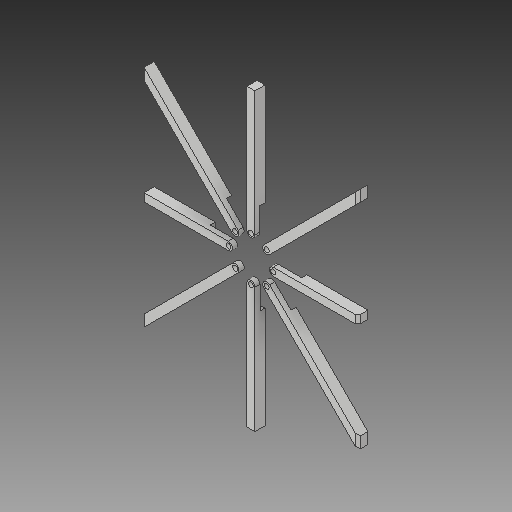
# Autodesk Inventor part: pins
Saved by Autodesk Inventor 2018.1 (Build 221171000, 171)
## iProperties
Created: 2017-08-02
Part Number: pins
Material: Generic
Document SubType Name: Modeling
Designer: Kai
Density: 1 g/cm^3
Appearance: Default
Author: Kai
Autodesk Inventor part; units mm, degrees
ref_plane "YZ Plane" through (0, 0, 0) normal (1, 0, 0) x (0, 1, 0)
ref_plane "XZ Plane" through (0, 0, 0) normal (0, 1, 0) x (-1, 0, 0)
ref_plane "XY Plane" through (0, 0, 0) normal (0, 0, 1) x (1, 0, 0)
sketch "Sketch1" plane through (0, 0, 0) normal (0, 0, 1) x (1, 0, 0)
  line L0 (0, 0) -> (0, 355.6) construction
  line L1 (-254, 0) -> (0, 0) construction
  line L2 (0, 355.6) -> (-254, 0) construction
  circle A0 centre (-127, 177.8) radius 38.1 construction
  circle A1 centre (-127, 177.8) radius 27.94 construction
  line L3 (0, 355.6) -> (0, 325.12) construction
  line L4 (-127, 177.8) -> (-100.0592, 204.7408) construction
  line L5 (-127, 177.8) -> (-95.96, 177.8) construction
  circle A2 centre (-107.2434, 197.5566) radius 3.1 construction
  circle A3 centre (-127, 205.74) radius 3.1 construction
  circle A4 centre (-127, 177.8) radius 27.94 construction
  circle A5 centre (-146.7566, 197.5566) radius 3.1 construction
  circle A6 centre (-127, 177.8) radius 27.94 construction
  circle A7 centre (-154.94, 177.8) radius 3.1 construction
  circle A8 centre (-127, 177.8) radius 27.94 construction
  circle A9 centre (-146.7566, 158.0434) radius 3.1 construction
  circle A10 centre (-127, 177.8) radius 27.94 construction
  circle A11 centre (-127, 149.86) radius 3.1 construction
  circle A12 centre (-127, 177.8) radius 27.94 construction
  circle A13 centre (-107.2434, 158.0434) radius 3.1 construction
  circle A14 centre (-127, 177.8) radius 27.94 construction
  circle A15 centre (-99.06, 177.8) radius 3.1 construction
  circle A16 centre (-127, 177.8) radius 27.94 construction
  arc A17 (-99.06, 182.8) -> (-98.6126, 172.8201) centre (-99.06, 177.8) ccw construction
  line L6 (-99.06, 182.8) -> (104.14, 182.8) construction
  line L7 (104.14, 182.8) -> (104.773, 172.8201) construction
  line L8 (104.773, 172.8201) -> (-99.5074, 172.8201) construction
  line L9 (-110.779, 201.0921) -> (32.9051, 344.7762) construction
  line L10 (32.9051, 344.7762) -> (40.4096, 338.1669) construction
  line L11 (40.4096, 338.1669) -> (-104.0384, 193.7189) construction
  arc A18 (-110.779, 201.0921) -> (-103.4057, 194.3516) centre (-107.2434, 197.5566) ccw construction
  line L12 (-132, 205.74) -> (-132, 408.94) construction
  line L13 (-132, 408.94) -> (-122.0201, 409.573) construction
  line L14 (-122.0201, 409.573) -> (-122.0201, 205.2926) construction
  arc A19 (-132, 205.74) -> (-122.0201, 206.1874) centre (-127, 205.74) ccw construction
  line L15 (-150.2921, 194.021) -> (-293.9762, 337.7051) construction
  line L16 (-293.9762, 337.7051) -> (-287.3669, 345.2096) construction
  line L17 (-287.3669, 345.2096) -> (-142.9189, 200.7616) construction
  arc A20 (-150.2921, 194.021) -> (-143.5516, 201.3943) centre (-146.7566, 197.5566) ccw construction
  line L18 (-154.94, 172.8) -> (-358.14, 172.8) construction
  line L19 (-358.14, 172.8) -> (-358.773, 182.7799) construction
  line L20 (-358.773, 182.7799) -> (-154.4926, 182.7799) construction
  arc A21 (-154.94, 172.8) -> (-155.3874, 182.7799) centre (-154.94, 177.8) ccw construction
  line L21 (-143.221, 154.5079) -> (-286.9051, 10.8238) construction
  line L22 (-286.9051, 10.8238) -> (-294.4096, 17.4331) construction
  line L23 (-294.4096, 17.4331) -> (-149.9616, 161.8811) construction
  arc A22 (-143.221, 154.5079) -> (-150.5943, 161.2484) centre (-146.7566, 158.0434) ccw construction
  line L24 (-122, 149.86) -> (-122, -53.34) construction
  line L25 (-122, -53.34) -> (-131.9799, -53.973) construction
  line L26 (-131.9799, -53.973) -> (-131.9799, 150.3074) construction
  arc A23 (-122, 149.86) -> (-131.9799, 149.4126) centre (-127, 149.86) ccw construction
  line L27 (-103.7079, 161.579) -> (39.9762, 17.8949) construction
  line L28 (39.9762, 17.8949) -> (33.3669, 10.3904) construction
  line L29 (33.3669, 10.3904) -> (-111.0811, 154.8384) construction
  arc A24 (-103.7079, 161.579) -> (-110.4484, 154.2057) centre (-107.2434, 158.0434) ccw construction
  line L30 (0, 355.6) -> (-254, 355.6) construction
  line L31 (-254, 0) -> (-254, 355.6) construction
  line L32 (-254, 355.6) -> (0, 355.6) construction
  line L33 (0, 355.6) -> (0, 0) construction
  line L34 (-254, 0) -> (0, 0) construction
  line L35 (-131.9799, -6.3504) -> (-122, -6.3494)
  line L36 (-122.0201, 361.9374) -> (-132, 361.9364)
  line L37 (-99.06, 182.8) -> (6.351, 182.8)
  line L38 (6.351, 182.8) -> (6.351, 172.8201)
  line L39 (6.351, 172.8201) -> (-99.5074, 172.8201)
  line L40 (-103.7079, 161.579) -> (6.3381, 51.533)
  line L41 (-110.4484, 154.2057) -> (6.3485, 37.4088)
  line L42 (-122, 149.86) -> (-122, -6.3494)
  line L43 (-131.9799, -6.3504) -> (-131.9799, 149.4126)
  arc A25 (-122, 149.86) -> (-131.9799, 149.4126) centre (-127, 149.86) ccw
  arc A26 (-103.7079, 161.579) -> (-110.4484, 154.2057) centre (-107.2434, 158.0434) ccw
  arc A27 (-99.06, 182.8) -> (-99.5074, 172.8201) centre (-99.06, 177.8) ccw
  circle A28 centre (-127, 149.86) radius 3.1
  circle A29 centre (-107.2434, 158.0434) radius 3.1
  circle A30 centre (-99.06, 177.8) radius 3.1
  circle A31 centre (-107.2434, 197.5566) radius 3.1
  arc A32 (-110.779, 201.0921) -> (-103.4057, 194.3516) centre (-107.2434, 197.5566) ccw
  circle A33 centre (-127, 205.74) radius 3.1
  arc A34 (-132, 205.74) -> (-122.0201, 206.1874) centre (-127, 205.74) ccw
  circle A35 centre (-146.7566, 197.5566) radius 3.1
  arc A36 (-150.2921, 194.021) -> (-142.9189, 200.7616) centre (-146.7566, 197.5566) ccw
  circle A37 centre (-154.94, 177.8) radius 3.1
  arc A38 (-154.94, 172.8) -> (-155.3874, 182.7799) centre (-154.94, 177.8) ccw
  circle A39 centre (-146.7566, 158.0434) radius 3.1
  arc A40 (-143.221, 154.5079) -> (-149.9616, 161.8811) centre (-146.7566, 158.0434) ccw
  line L44 (-154.94, 172.8) -> (-260.35, 172.8)
  line L45 (-154.4926, 182.7799) -> (-260.35, 182.7799)
  line L46 (6.3485, 37.4088) -> (6.3381, 51.533)
  line L47 (-143.221, 154.5079) -> (-260.35, 37.3789)
  line L48 (-260.35, 51.4927) -> (-150.293, 161.5781)
  line L49 (-150.293, 161.5781) -> (-149.9616, 161.8811)
  line L50 (-260.35, 51.4927) -> (-260.35, 37.3789)
  line L51 (-142.9189, 200.7616) -> (-260.35, 318.1927)
  line L52 (-260.35, 304.0789) -> (-150.2921, 194.021)
  line L53 (-132, 361.9364) -> (-132, 205.74)
  line L54 (-122.0201, 206.1874) -> (-122.0201, 361.9374)
  line L55 (6.351, 304.1083) -> (-103.4057, 194.3516)
  line L56 (6.351, 318.2221) -> (-110.779, 201.0921)
  line L57 (-260.35, 318.1927) -> (-260.35, 304.0789)
  line L58 (-260.35, 182.7799) -> (-260.35, 172.8)
  line L59 (6.351, 172.8201) -> (6.351, 182.8)
  line L60 (6.351, 304.1083) -> (6.351, 318.2221)
  dimension "d4" = 76.2
  dimension "d5" = 55.88
  dimension "d6" = 30.48
  dimension "d7" = 45
  dimension "d8" = 6.2
  dimension "d9" = 360
  dimension "d10" = 10
  dimension "d11" = 203.2
  dimension "d12" = 10
  dimension "d13" = 360
  constraints: 122 end point, 48 point on circle, 33 centre point, 27 point on line, 20 coincident, 15 concentric, 4 coincident with centre, 3 collinear, 3 perpendicular, 3 tangent, 2 horizontal alignment, 2 vertical alignment, 1 midpoint, 1 parallel, 129 other
  measures "d6" distance of L3.start L3.end
  measures "d7" angle of L5 L4
  measures "d8" diameter of A2
  measures "d10" diameter of A17
  measures "d11" distance of L37.start L6.end
  measures "d12" distance of L6.end L7.end
extrude "Extrusion1" add sketch "Sketch1" along normal blind 12.7
sketch "Sketch2" plane through (0, 0, 0) normal (0, 0, -1) x (-1, 0, 0)
  circle A0 centre (146.7566, 197.5566) radius 3.1 construction
  circle A1 centre (107.2434, 158.0434) radius 3.1 construction
  line L0 (146.7566, 197.5566) -> (107.2434, 158.0434) construction
  circle A2 centre (127, 177.8) radius 57.15
  point P0 (0, 0)
  dimension "d17" = 114.3
  constraints: 2 end point, 1 centre point, 1 midpoint
  measures "d17" diameter of A2
extrude "Extrusion2" cut sketch "Sketch2" against normal blind 6.35
sketch "Sketch3" plane through (-99.5074, 172.8201, 12.7) normal (0, -1, 0) x (1, 0, 0)
  line L0 (102.6704, 0) -> (105.8454, -3.175)
  line L1 (106.7063, 0) -> (102.6704, 0)
  line L2 (106.7063, 0) -> (105.8454, -3.175)
  point P0 (99.5074, -12.7)
  point P1 (105.8454, 0)
  constraints: 6 end point, 1 horizontal
extrude "Extrusion3" cut sketch "Sketch3" along normal mid plane 508
body "Solid1"
